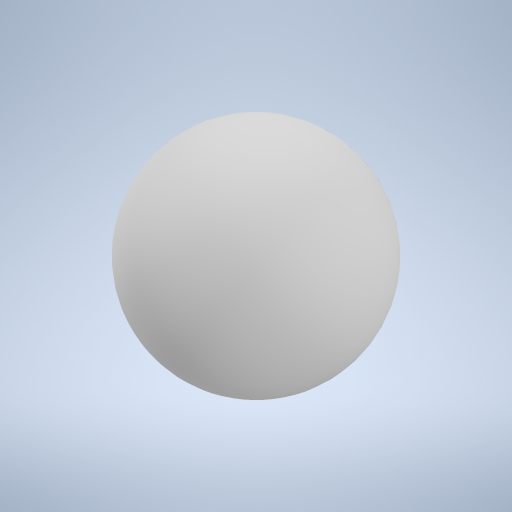
# Autodesk Inventor part: HUNDSON-1-44
Saved by Autodesk Inventor 2024.2 (Build 282272000, 272)
## iProperties
Created: 2024-10-10
Part Number: HUNDSON-1-44
Material: Generic
Document SubType Name: Modeling
Designer: Precisión-05
Density: 1 g/cm^3
Appearance: Default
Author: Precisión-05
Autodesk Inventor part; units mm, degrees
ref_plane "YZ Plane" through (0, 0, 0) normal (1, 0, 0) x (0, 1, 0)
ref_plane "XZ Plane" through (0, 0, 0) normal (0, 1, 0) x (-1, 0, 0)
ref_plane "XY Plane" through (0, 0, 0) normal (0, 0, 1) x (1, 0, 0)
sketch "Sketch1" plane through (0, 0, 0) normal (0, 0, 1) x (1, 0, 0)
  line L0 (-4.9166, -5.0979) -> (-4.9166, -1.0979)
  arc A0 (-4.9166, -1.0979) -> (-4.9166, -9.0979) centre (-4.9166, -5.0979) ccw
  line L1 (-4.9166, -5.0979) -> (-4.9166, -9.0979)
  point P0 (0, 0)
  dimension "d0" = 4
  constraints: 4 end point, 2 point on circle, 2 vertical, 1 centre point, 1 coincident
  measures "d0" distance of L0.start L0.end
revolve "Revolution1" add sketch "Sketch1" angle 360 about axis through (-4.9166, -5.0979, 0) along (0, -1, 0)
body "Solid1"
